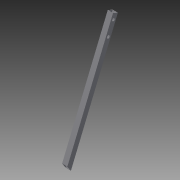
# Autodesk Inventor part: CatapultArmSquare-Top
Saved by Autodesk Inventor 2013 (Build 170138000, 138)
## iProperties
Created: 2014-01-20
Part Number: CatapultArmSquare-Top
Material: Generic
Document SubType Name: Modeling
Designer: RobertB
Density: 1 g/cm^3
Author: RobertB
Autodesk Inventor part; units mm, degrees
ref_plane "YZ Plane" through (0, 0, 0) normal (1, 0, 0) x (0, 1, 0)
ref_plane "XZ Plane" through (0, 0, 0) normal (0, 1, 0) x (-1, 0, 0)
ref_plane "XY Plane" through (0, 0, 0) normal (0, 0, 1) x (1, 0, 0)
sketch "Sketch1" plane through (0, 0, 0) normal (1, 0, 0) x (0, 1, 0)
  line L0 (0, 0) -> (0, 254)
  line L1 (0, 0) -> (254, 0) construction
  line L2 (0, 0) -> (527.9972, -218.7036)
  line L3 (0, 0) -> (571.5, 0) construction
  line L4 (0, 254) -> (-25.4, 254)
  line L5 (0, 254) -> (25.4, 254) construction
  line L6 (527.9972, -218.7036) -> (518.277, -242.1701)
  line L7 (527.9972, -218.7036) -> (553.3972, -218.7036) construction
  line L8 (518.277, -242.1701) -> (-25.4, -16.9717)
  line L9 (-25.4, -16.9717) -> (-25.4, 254)
  line L10 (-25.4, -16.9717) -> (0, 0)
  dimension "d0" = 254
  dimension "d1" = 90
  dimension "d2" = 571.5
  dimension "d3" = 22.5
  dimension "d4" = 25.4
  dimension "d5" = 180
  dimension "d6" = 25.4
  dimension "d7" = 112.5
  dimension "d8" = 90
  constraints: 22 end point, 4 equal length, 4 horizontal, 2 perpendicular, 1 parallel, 1 vertical
  measures "d0" distance of L0.start L0.end
  measures "d1" angle of L1 L0
  measures "d2" distance of L0.start L2.end
  measures "d3" angle of L2 L3
  measures "d4" distance of L0.end L4.end
  measures "d5" angle of L4 L5
  measures "d6" distance of L2.end L6.end
  measures "d7" angle of L6 L7
  measures "d8" angle of L6 L8
extrude "Extrusion3" add sketch "Sketch1" along normal blind 25.4 contours L2 L6 L8 L10
sketch "Sketch3" plane through (0, 527.9972, -218.7036) normal (0, 0.9239, -0.3827) x (1, 0, 0)
  line L0 (0, 25.4) -> (1.5875, 25.4)
  line L1 (1.5875, 25.4) -> (1.5875, 23.8125)
  line L2 (1.5875, 23.8125) -> (0, 23.8125)
  line L3 (0, 23.8125) -> (0, 25.4)
  line L4 (25.4, 0) -> (23.8125, 0)
  line L5 (23.8125, 0) -> (23.8125, 1.5875)
  line L6 (23.8125, 1.5875) -> (25.4, 1.5875)
  line L7 (25.4, 1.5875) -> (25.4, 0)
  line L8 (1.5875, 23.8125) -> (23.8125, 23.8125)
  line L9 (23.8125, 23.8125) -> (23.8125, 1.5875)
  line L10 (23.8125, 1.5875) -> (1.5875, 1.5875)
  line L11 (1.5875, 1.5875) -> (1.5875, 23.8125)
  dimension "d19" = 1.5875
  dimension "d20" = 1.5875
  dimension "d21" = 1.5875
  dimension "d22" = 1.5875
  constraints: 24 end point, 6 parallel, 3 horizontal, 3 perpendicular
  measures "d19" distance of L1.end L2.end
  measures "d20" distance of L0.end L1.end
  measures "d21" distance of L5.end L6.end
  measures "d22" distance of L4.end L5.end
extrude "Extrusion4" cut sketch "Sketch3" against normal blind 2540 contours L8 L9 L10 L11
sketch "Sketch4" plane through (25.4, 0, 0) normal (1, 0, 0) x (0, 0, -1)
  line L0 (242.1701, 518.277) -> (218.7036, 527.9972) projected
  line L1 (218.7036, 527.9972) -> (0, 0) projected
  line L2 (230.4369, 523.1371) -> (220.7167, 499.6705)
  line L3 (230.4369, 523.1371) -> (255.8369, 523.1371) construction
  circle A0 centre (220.7167, 499.6705) radius 6.35
  line L4 (220.7167, 499.6705) -> (196.4163, 441.0042)
  circle A1 centre (196.4163, 441.0042) radius 7.112
  dimension "d25" = 25.4
  dimension "d26" = 112.5
  dimension "d27" = 12.7
  dimension "d28" = 63.5
  dimension "d29" = 14.224
  constraints: 6 end point, 2 centre point, 2 coincident, 1 collinear, 1 equal length, 1 horizontal, 1 midpoint, 1 parallel
  measures "d25" distance of L2.start L2.end
  measures "d26" angle of L2 L3
  measures "d27" diameter of A0
  measures "d28" distance of L4.start L4.end
  measures "d29" diameter of A1
extrude "Extrusion5" cut sketch "Sketch4" against normal blind 50.8
body "Solid2"
